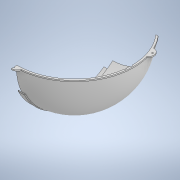
# Autodesk Inventor part: dome
Saved by Autodesk Inventor 2021 (Build 250183000, 183)
## iProperties
Created: 2020-05-29
Part Number: dome
Material: Generic
Document SubType Name: Modeling
Designer: Daniel
Density: 1 g/cm^3
Appearance: Default
Author: Daniel
Autodesk Inventor part; units mm, degrees
ref_plane "YZ Plane" through (0, 0, 0) normal (1, 0, 0) x (0, 1, 0)
ref_plane "XZ Plane" through (0, 0, 0) normal (0, 1, 0) x (-1, 0, 0)
ref_plane "XY Plane" through (0, 0, 0) normal (0, 0, 1) x (1, 0, 0)
sketch "Sketch1" plane through (0, 0, 0) normal (1, 0, 0) x (0, 1, 0)
  line L0 (0, 0) -> (19.0301, 0) construction
  circle A0 centre (150, 0) radius 150
  circle A1 centre (150, 0) radius 152
  line L1 (150, 0) -> (150, 152)
  line L2 (150, 152) -> (150, 167)
  line L3 (150, 167) -> (153, 167)
  line L4 (153, 167) -> (153, 151.9704)
  line L5 (0, 0) -> (-2, 0)
  line L6 (153, 151.9704) -> (153, 150)
  line L7 (153, 150) -> (150, 150)
  line L8 (153, 150.4) -> (150, 150.4)
  point P0 (150, 150)
  dimension "d3" = 300
  dimension "d4" = 2
  dimension "d5" = 15
  dimension "d30" = 3
  dimension "d40" = 0.4
  constraints: 18 end point, 6 point on line, 5 point on circle, 4 perpendicular, 2 centre point, 2 vertical, 1 horizontal
  measures "d3" diameter of A0
  measures "d4" radial gap between concentric circles of A0 A1
  measures "d5" distance of L1.end L2.end
  measures "d30" distance of L2.end L3.end
  measures "d40" distance between parallel lines of L7 L8
revolve "Revolution1" add sketch "Sketch1" angle 360 about axis through (0, 0, 0) along (0, 1, 0) contours A0 L5 A1 L1 | L1 A1 L6 L8 | L2 L3 L4 A1
sketch "Sketch2" plane through (0, 153, 0) normal (0, 1, 0) x (1, 0, 0)
  line L0 (-160.6894, 100) -> (177.2685, 100)
  line L1 (177.2685, 100) -> (177.2685, 219.2417)
  line L2 (177.2685, 219.2417) -> (-160.6894, 219.2417)
  line L3 (-160.6894, 219.2417) -> (-160.6894, 100)
  point P0 (0, 0)
  dimension "d8" = 100
  constraints: 8 end point, 2 parallel, 1 horizontal, 1 perpendicular
  measures "d8" distance from line of point (0, 0) L0
extrude "Extrusion1" cut sketch "Sketch2" against normal through all
split "Split1" plane through (0, 0, 0) removes the side toward (-1, 0, 0)
sketch "Sketch3" plane through (111.8034, 153, -100) normal (0, 1, 0) x (1, 0, 0)
  circle A0 centre (-111.8034, -259) radius 2.1
  circle A1 centre (37.6077, -45.6188) radius 2.1
  circle A2 centre (37.6077, -45.6188) radius 6
  circle A3 centre (-111.8034, -259) radius 6
  line L0 (-111.8034, -100) -> (37.6077, -45.6188) construction
  arc A4 (-111.8034, -255) -> (-47.3258, 40.9526) centre (-111.8034, -100) ccw
  arc A5 (38.2956, -61.3311) -> (28.035, -33.1403) centre (28.351, -48.988) ccw
  arc A6 (-111.8034, -265) -> (-96.8034, -254.2725) centre (-111.8034, -249.1492) ccw
  arc A7 (-111.8034, -252) -> (2.6693, 0) centre (-111.8034, -100) ccw construction
  arc A8 (-111.8034, -335) -> (-14.047, 113.7023) centre (-111.8034, -100) ccw
  line L1 (-14.047, 113.7023) -> (-47.3258, 40.9526)
  line L2 (-111.8034, -335) -> (-111.8034, -255)
  line L3 (-111.8034, -250.4) -> (-111.8034, -267) construction
  line L4 (-111.8034, 0) -> (-111.8034, -250) construction
  point P0 (-111.8034, -256.9)
  point P1 (-111.8034, -261.1)
  point P2 (33.849, -46.9869)
  dimension "d14" = 12
  dimension "d11" = 4.2
  dimension "d20" = 15
  dimension "d21" = 15
  dimension "d32" = 3
  dimension "d33" = 110
  dimension "d35" = 15
  dimension "d60" = 4
  dimension "d61" = 4
  dimension "d62" = 80
  constraints: 12 point on circle, 7 centre point, 6 end point, 3 coincident, 3 point on line, 2 collinear, 1 concentric, 1 equal radius, 1 line through centre, 1 tangent, 5 other
  measures "d11" diameter of A0
  measures "d20" distance from line of A5.end L0
  measures "d21" distance from line of L0 A5.start
  measures "d32" radial gap between concentric circles of A7 A4
  measures "d33" angle of L4 L0
  measures "d35" distance from line of L3 A6.end
  measures "d60" distance of A0.centre L2.end
  measures "d61" distance of A1.centre point (33.849, -46.987)
  measures "d62" distance of L1.start L1.end
extrude "Extrusion2" cut sketch "Sketch3" against normal through all contours A0 L2 | L2 A0 | A6 A4 A5 L1 A8 L2 | A1
sketch "Sketch4" plane through (0, 153, 0) normal (0, 1, 0) x (0.9128709, 0, 0.4082483)
  line L0 (0, 0) -> (114.0893, 51.0223)
  circle A0 centre (137.9322, 58.9466) radius 2.5
  circle A1 centre (143.1399, 44.8438) radius 2.5
  arc A2 (61.4005, -137.2958) -> (61.7266, 137.1495) centre (0, 0) ccw construction
  arc A3 (61.2372, -136.9306) -> (61.2372, 136.9306) centre (0, 0) ccw construction
  line L1 (-40.8248, 91.2871) -> (61.2372, -136.9306) construction
  dimension "d23" = 5
  dimension "d24" = 5
  dimension "d25" = 2.5
  dimension "d26" = 17.5
  dimension "d59" = 90
  constraints: 2 centre point, 2 end point, 3 other
  measures "d23" diameter of A0
  measures "d24" diameter of A1
  measures "d25" distance from line of L0 A0.centre
  measures "d26" distance from line of A1.centre L0
  measures "d59" angle of L1 L0
extrude "Extrusion3" cut sketch "Sketch4" against normal blind 2
sketch "Sketch5" plane through (0, 0, 0) normal (0, 0, 1) x (1, 0, 0)
  arc A0 (0, -2) -> (152, 150) centre (0, 150) ccw construction
  line L0 (0, 150) -> (-144.4306, 150) construction
  arc A1 (-10, -1.6707) -> (10, -1.6707) centre (0, 150) ccw
  line L1 (10, -1.6707) -> (10, -3.6707)
  line L2 (-10, -1.6707) -> (-10, -3.6707)
  arc A2 (-10, -3.6707) -> (10, -3.6707) centre (0, 149.0011) ccw
  point P0 (0, 0)
  dimension "d41" = 20
  dimension "d42" = 10
  dimension "d43" = 2
  dimension "d44" = 2
  constraints: 7 point on circle, 6 end point, 2 centre point, 2 vertical, 1 horizontal, 1 tangent
  measures "d41" distance of L1.start L2.start
  measures "d42" horizontal distance of A0.start L1.start
  measures "d43" distance of L1.start L1.end
  measures "d44" distance of L2.start L2.end
revolve "Revolution2" add sketch "Sketch5" angle 65 about axis through (0, 150, 0) along (-1, 0, 0) and the other way 35
chamfer "Chamfer1" distance 2 angle 45 2 edges at (10, 1.5655, 39.7729) (-10, 1.5655, 39.7729)
equation "\"d21\" = d20"
equation "\"d44\" = d43"
body "Solid1"
